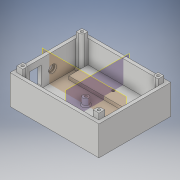
# Autodesk Inventor part: Masterboxbottom
Saved by Autodesk Inventor 2019 (Build 230136000, 136)
## iProperties
Created: 2019-08-02
Part Number: Masterboxbottom
Material: Generic
Document SubType Name: Modeling
Designer: Riley
Density: 1 g/cm^3
Appearance: Default
Author: Riley
Autodesk Inventor part; units mm, degrees
ref_plane "YZ Plane" through (0, 0, 0) normal (1, 0, 0) x (0, 1, 0)
ref_plane "XZ Plane" through (0, 0, 0) normal (0, 1, 0) x (-1, 0, 0)
ref_plane "XY Plane" through (0, 0, 0) normal (0, 0, 1) x (1, 0, 0)
sketch "Sketch1" plane through (0, 0, 0) normal (0, 1, 0) x (-1, 0, 0)
  line L0 (0, 0) -> (89.5858, 0)
  line L1 (89.5858, 0) -> (89.5858, 71.12)
  line L2 (89.5858, 71.12) -> (0, 71.12)
  line L3 (0, 71.12) -> (0, 0)
  line L4 (-3.556, -3.556) -> (93.1418, -3.556)
  line L5 (93.1418, -3.556) -> (93.1418, 74.676)
  line L6 (93.1418, 74.676) -> (-3.556, 74.676)
  line L7 (-3.556, 74.676) -> (-3.556, -3.556)
  dimension "d0" = 89.5858
  dimension "d1" = 71.12
  dimension "d2" = 3.556
  dimension "d3" = 3.556
  dimension "d4" = 3.556
  dimension "d5" = 3.556
  constraints: 16 end point, 4 parallel, 2 horizontal, 2 perpendicular
  measures "d0" distance of L2.end L1.end
  measures "d1" distance of L1.end L0.end
  measures "d2" distance between parallel lines of L1 L5
  measures "d3" distance between parallel lines of L2 L6
  measures "d4" distance between parallel lines of L3 L7
  measures "d5" distance between parallel lines of L4 L0
extrude "Extrusion1" add sketch "Sketch1" along normal blind 28.4226
sketch "Sketch2" plane through (0, 0, 0) normal (0, -1, 0) x (1, 0, 0)
  line L0 (-93.1418, 74.676) -> (3.556, 74.676) projected
  line L1 (3.556, 74.676) -> (-93.1418, 74.676)
  line L2 (-93.1418, 74.676) -> (-93.1418, -3.556)
  line L3 (-93.1418, -3.556) -> (3.556, -3.556)
  line L4 (3.556, -3.556) -> (3.556, 74.676)
  line L5 (0, 0) -> (0, 71.12) projected
  dimension "d61" = 93.1418
  dimension "d75" = 78.232
  constraints: 8 end point, 2 parallel, 1 horizontal, 1 perpendicular
  measures "d61" distance between parallel lines of L5 L2
  measures "d75" distance between parallel lines of L0 L3
extrude "Extrusion2" add sketch "Sketch2" along normal blind 3.556
sketch "Sketch8" plane through (0, 0, 0) normal (0, 1, 0) x (1, 0, 0)
  circle A0 centre (-6.3627, -55.9054) radius 1.2827
  line L0 (0, 0) -> (0, -71.12) projected
  line L1 (0, -71.12) -> (-89.5858, -71.12) projected
  line L2 (-6.3627, -55.9054) -> (-50.2539, -55.9054)
  line L3 (-50.2539, -55.9054) -> (-50.2539, -35.1028)
  line L4 (-50.2539, -35.1028) -> (-6.3627, -35.1028)
  line L5 (-6.3627, -35.1028) -> (-6.3627, -55.9054)
  circle A1 centre (-6.3627, -55.9054) radius 3.2258
  dimension "d32" = 2.5654
  dimension "d33" = 6.3627
  dimension "d34" = 15.2146
  dimension "d35" = 43.8912
  dimension "d36" = 20.8026
  dimension "d45" = 6.4516
  constraints: 8 end point, 2 centre point, 2 parallel, 1 coincident, 1 horizontal, 1 perpendicular
  measures "d32" diameter of A0
  measures "d33" distance from line of L0 L2.start
  measures "d34" distance from line of L1 L2.start
  measures "d35" distance of L3.end L4.end
  measures "d36" distance between parallel lines of L2 L4
  measures "d45" diameter of A1
extrude "Extrusion8" add sketch "Sketch8" along normal blind 7.62 contours A0 L5 A1 L2 | A0 L2 A1 L5
pattern_linear "Rectangular Pattern2" count 2 spacing 43.8912 along (-1, 0, 0) count 2 spacing -20.8026 along (0, 0, 1) of "Extrusion8"
chamfer "Chamfer2" distance 1.27 angle 45 4 edges at (-9.5885, 0, 55.9054) (-53.4797, 0, 55.9054) (-53.4797, 0, 35.1028) (-9.5885, 0, 35.1028)
sketch "Sketch11" plane through (-93.1418, 28.4226, -3.556) normal (-1, 0, 0) x (0, 0, 1)
  circle A0 centre (35.56, -15.9893) radius 3.1369
  line L0 (78.232, -31.9786) -> (0, -31.9786) projected
  line L1 (0, -28.4226) -> (0, 0) projected
  line L2 (47.9044, -6.35) -> (60.452, -6.35)
  line L3 (60.452, -6.35) -> (60.452, -25.6286)
  line L4 (60.452, -25.6286) -> (47.9044, -25.6286)
  line L5 (47.9044, -25.6286) -> (47.9044, -6.35)
  line L6 (78.232, -31.9786) -> (78.232, 0) projected
  line L7 (0, 0) -> (78.232, 0) projected
  point P0 (3.556, -28.4226)
  point P1 (62.992, -28.4226)
  dimension "d63" = 6.2738
  dimension "d64" = 15.9893
  dimension "d65" = 35.56
  dimension "d66" = 12.5476
  dimension "d67" = 19.2786
  dimension "d68" = 17.78
  dimension "d69" = 6.35
  dimension "d71" = 31.9786
  constraints: 8 end point, 2 parallel, 1 centre point, 1 horizontal, 1 perpendicular, 1 other
  measures "d63" diameter of A0
  measures "d64" distance from line of L0 A0.centre
  measures "d65" distance from line of L1 A0.centre
  measures "d66" distance of L3.end L4.end
  measures "d67" distance of L2.end L3.end
  measures "d69" distance between parallel lines of L7 L2
  measures "d71" distance between parallel lines of L0 L7
extrude "Extrusion9" cut sketch "Sketch11" along normal mid plane 25.4
ref_plane "Work Plane5" through (-44.7929, 28.4226, -3.556) normal (-1, 0, 0) x (0, 0, 1)
ref_plane "Work Plane6" through (-93.1418, 28.4226, 35.56) normal (0, 0, 1) x (1, 0, 0)
sketch "Sketch18" plane through (0, 0, 0) normal (0, 1, 0) x (1, 0, 0)
  circle A0 centre (-3.2829, -3.283) radius 1.505
  arc A1 (-6.5659, -3.283) -> (-3.2829, -6.5659) centre (-3.2829, -3.283) ccw
  line L0 (-89.5858, 0) -> (0, 0) projected
  line L1 (0, 0) -> (0, -71.12) projected
  line L2 (-6.5659, -3.283) -> (-6.5659, 0)
  line L3 (-3.2829, -6.5659) -> (0, -6.5659)
  line L4 (0, -71.12) -> (0, 0) projected
  line L5 (0, 0) -> (0, -6.5659)
  line L6 (0, 0) -> (-6.5659, 0)
  point P0 (0, -7.2625)
  point P1 (0, -6.4624)
  dimension "d105" = 3.0099
  dimension "d106" = 6.5659
  constraints: 8 end point, 2 centre point, 2 collinear, 2 perpendicular, 2 point on circle, 2 point on line, 2 tangent, 1 coincident
  measures "d105" diameter of A0
  measures "d106" diameter of A1
extrude "Extrusion12" add sketch "Sketch18" along normal blind 34.7726
mirror "Mirror9" about plane through (-93.1418, 28.4226, 35.56) normal (0, 0, 1) of "Extrusion12"
mirror "Mirror10" about plane through (-44.7929, 28.4226, -3.556) normal (-1, 0, 0) of "Extrusion12", "Mirror9"
chamfer "Chamfer3" distance 2.032 angle 45 11 edges at (-6.5659, 0, 69.4785) (-5.6043, 0, 65.5157) (-1.6415, 0, 64.5541) (-6.5659, 0, 1.6415) (-5.6043, 0, 5.6043) (-83.9815, 0, 65.5157) (-83.0199, 0, 69.4785) (-87.9443, 0, 64.5541) (-83.9815, 0, 5.6043) (-87.9443, 0, 6.5659) (-83.0199, 0, 1.6415)
sketch "Sketch22" plane through (-89.5858, 28.4226, 64.5541) normal (1, 0, 0) x (0, 0, -1)
  circle A0 centre (32.5501, -15.9893) radius 3.1369 projected
  circle A1 centre (32.5501, -15.9893) radius 4.318
  point P0 (64.5541, -28.4226)
  dimension "d125" = 8.636
  constraints: 1 centre point, 1 coincident
  measures "d125" diameter of A1
extrude "Extrusion13" cut sketch "Sketch22" against normal blind 1.778
thicken "Thicken1" operation cut thickness 0.2032 both sides no extend neighbours no toward (0, 0, 1) faces at (-2.1886, 30.5393, 0)
thicken "Thicken2" operation cut thickness 0.2032 both sides no extend neighbours no toward (1, 0, 0) faces at (0, 32.6559, 66.7427)
thicken "Thicken3" operation cut thickness 0.2032 both sides no extend neighbours no toward (1, 0, 0) faces at (0, 30.5393, 4.445)
thicken "Thicken4" operation cut thickness 0.2032 both sides no extend neighbours no toward (-1, 0, 0) faces at (0, 30.5393, 4.445)
thicken "Thicken5" operation cut thickness 0.2032 both sides no extend neighbours no toward (0, 0, 1) faces at (-87.3972, 32.6559, 0)
thicken "Thicken6" operation cut thickness 0.2032 both sides no extend neighbours no toward (1, 0, 0) faces at (-89.5858, 30.5393, 4.445)
thicken "Thicken7" operation cut thickness 0.2032 both sides no extend neighbours no toward (1, 0, 0) faces at (-89.5858, 32.6559, 66.7427)
thicken "Thicken8" operation cut thickness 0.2032 both sides no extend neighbours no toward (0, 0, -1) faces at (-85.1408, 32.6559, 71.12)
thicken "Thicken9" operation cut thickness 0.2032 both sides no extend neighbours no toward (0, 0, -1) faces at (-2.1886, 30.5393, 71.12)
thicken "Thicken10" operation cut thickness 0.2032 both sides no extend neighbours no toward (-1, 0, 0) faces at (0, 32.6559, 68.7959)
sketch "Sketch24" plane through (0, 0, 0) normal (0, 1, 0) x (1, 0, 0)
  line L0 (-6.5659, 0) -> (-83.0199, 0)
  line L1 (-83.0199, 0) -> (-83.0199, -21.0312)
  line L2 (-83.0199, -21.0312) -> (-6.5659, -21.0312)
  line L3 (-6.5659, -21.0312) -> (-6.5659, 0)
  line L4 (-83.0199, 0) -> (-6.5659, 0) projected
  line L5 (-6.5659, -0.2032) -> (-6.5659, -3.283) projected
  dimension "d163" = 76.454
  dimension "d164" = 21.0312
  constraints: 8 end point, 2 collinear, 2 parallel, 1 horizontal, 1 perpendicular
  measures "d163" distance of L2.end L1.end
  measures "d164" distance of L1.end L0.end
extrude "Extrusion15" add sketch "Sketch24" along normal blind 3.556
sketch "Sketch25" plane through (0, 3.556, 0) normal (0, 1, 0) x (1, 0, 0)
  circle A0 centre (-44.7421, -10.795) radius 1.4224
  line L0 (-83.0199, -21.2344) -> (-6.5659, -21.2344) projected
  line L1 (-6.5659, -21.2344) -> (-6.5659, -3.283) projected
  point P0 (0, 0)
  dimension "d157" = 2.8448
  dimension "d158" = 10.4394
  dimension "d159" = 38.1762
  constraints: 1 centre point
  measures "d157" diameter of A0
  measures "d158" distance from line of L0 A0.centre
  measures "d159" distance from line of L1 A0.centre
extrude "Extrusion16" cut sketch "Sketch25" against normal blind 4.3688
ref_plane "Work Plane7" through (-44.7929, 28.4226, -3.556) normal (-1, 0, 0) x (0, 0, 1)
equation "\"d0\" = 2 * d106 + d153"
equation "\"d3\" = d2"
equation "\"d4\" = d2"
equation "\"d5\" = d2"
equation "\"d61\" = d0 + d2"
equation "\"d75\" = d1 + 2 * d2"
equation "\"d8\" = d2"
equation "\"d50\" = d35"
equation "\"d53\" = -d36"
equation "\"d64\" = 0.5 * d71"
equation "\"d68\" = 0.5 * d65"
equation "\"d69\" = -0.5 * d67 + 0.5 * d71"
equation "\"d126\" = 0.5 * d2"
equation "\"d98\" = -0.5 * d0 - d2"
equation "\"d99\" = -0.5 * d1 - d2"
equation "\"d153\" = 76.454"
body "Solid1"
